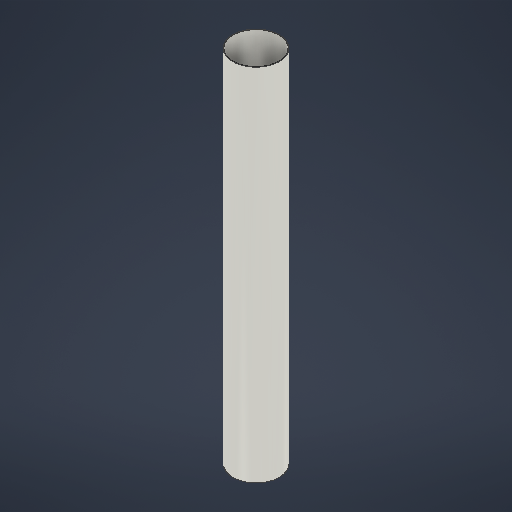
# Autodesk Inventor part: CAMARA_DE_COMBUSTION
Saved by Autodesk Inventor 2025 (Build 290162010, 162A)
## iProperties
Created: 2024-07-23
Part Number: CAMARA_DE_COMBUSTION
Material: Genérico
Document SubType Name: Modeling
Designer: hansm
Density: 1 g/cm^3
Appearance: Abedul - Natural pulido
Author: hansm
Autodesk Inventor part; units mm, degrees
ref_plane "YZ Plane" through (0, 0, 0) normal (1, 0, 0) x (0, 1, 0)
ref_plane "XZ Plane" through (0, 0, 0) normal (0, 1, 0) x (-1, 0, 0)
ref_plane "XY Plane" through (0, 0, 0) normal (0, 0, 1) x (1, 0, 0)
sketch "Boceto1" plane through (0, 0, 0) normal (0, 1, 0) x (-1, 0, 0)
  circle A0 centre (0, 0) radius 39
  circle A1 centre (0, 0) radius 38
  dimension "d0" = 78
  dimension "d1" = 76
  constraints: 2 centre point, 2 coincident
  measures "d0" diameter of A0
  measures "d1" diameter of A1
extrude "Extrusión1" add sketch "Boceto1" along normal blind 600
